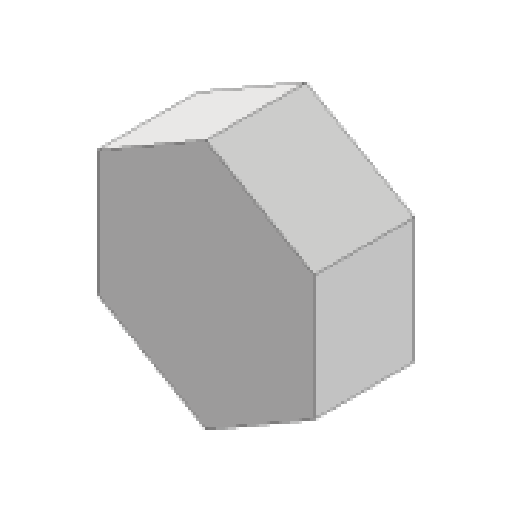
# Autodesk Inventor part: M3_nut
Saved by Autodesk Inventor 2023 (Build 270158000, 158)
## iProperties
Created: 2022-09-20
Part Number: M3_nut
Material: Generic
Document SubType Name: Modeling
Designer: CDT
Density: 1 g/cm^3
Appearance: Default
Author: CDT
Autodesk Inventor part; units mm, degrees
ref_plane "YZ Plane" through (0, 0, 0) normal (1, 0, 0) x (0, 1, 0)
ref_plane "XZ Plane" through (0, 0, 0) normal (0, 1, 0) x (-1, 0, 0)
ref_plane "XY Plane" through (0, 0, 0) normal (0, 0, 1) x (1, 0, 0)
sketch "Sketch1" plane through (0, 0, 0) normal (0, 0, 1) x (1, 0, 0)
  line L0 (0, -2.8) -> (-2.4249, -1.4)
  line L1 (-2.4249, -1.4) -> (-2.4249, 1.4)
  line L2 (-2.4249, 1.4) -> (0, 2.8)
  line L3 (0, 2.8) -> (2.4249, 1.4)
  line L4 (2.4249, 1.4) -> (2.4249, -1.4)
  line L5 (2.4249, -1.4) -> (0, -2.8)
  point P0 (0, 0)
  point P1 (0, 0)
  dimension "d0" = 2.8
  constraints: 12 end point, 1 coincident, 13 other
  measures "d0" distance of L0.start point (0, 0)
extrude "Extrusion1" add sketch "Sketch1" along normal blind 2
sketch "Sketch2" plane through (0, 0, 2) normal (0, 0, 1) x (1, 0, 0)
  circle A0 centre (0, 0) radius 1.5
  dimension "d3" = 3
  constraints: 1 centre point, 1 coincident
  measures "d3" diameter of A0
extrude "Extrusion2" cut sketch "Sketch2" against normal through all
body "Solid1"
